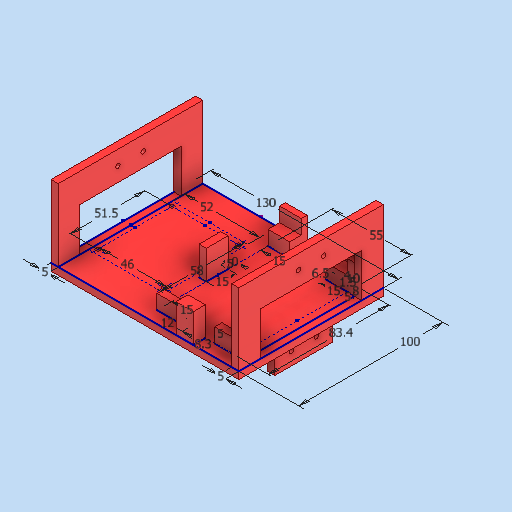
# Autodesk Inventor part: Chasis 2
Saved by Autodesk Inventor 2026.2 (Build 302298010, 298A)
## iProperties
Created: 2025-12-05
Part Number: Chasis 2
Material: Generic
Document SubType Name: Modeling
Designer: maxim
Density: 1 g/cm^3
Appearance: Light Red
Author: maxim
Autodesk Inventor part; units mm, degrees
ref_plane "YZ Plane" through (0, 0, 0) normal (1, 0, 0) x (0, 1, 0)
ref_plane "XZ Plane" through (0, 0, 0) normal (0, 1, 0) x (-1, 0, 0)
sketch "Sketch1" plane through (0, 0, 0) normal (0, 1, 0) x (-1, 0, 0)
  line L0 (0, 0) -> (-130, 0)
  line L1 (-130, 0) -> (-130, -100)
  line L2 (-130, -100) -> (0, -100)
  line L3 (0, -100) -> (0, 0)
  line L4 (-5, -21) -> (-57, -21) construction
  line L5 (-65, -21) -> (-65, -79) construction
  line L6 (-57, -79) -> (-5, -79) construction
  line L7 (-5, -79) -> (-5, -21) construction
  line L8 (-65, -91.7) -> (-120, -91.7) construction
  line L9 (-120, -91.7) -> (-120, -8.3) construction
  line L10 (-120, -8.3) -> (-65, -8.3) construction
  line L11 (-65, -8.3) -> (-65, -91.7) construction
  line L12 (-5, 0) -> (-5, -100)
  line L13 (-125, -100) -> (-125, 0)
  line L14 (-86.5, 0) -> (-98.5, 0)
  line L15 (-98.5, 0) -> (-98.5, -8.3)
  line L16 (-98.5, -8.3) -> (-86.5, -8.3)
  line L17 (-86.5, -8.3) -> (-86.5, 0)
  line L18 (-87.5, -100) -> (-97.5, -100)
  line L19 (-110, -93.2) -> (-120, -93.2)
  line L20 (-120, -93.2) -> (-120, -85.2)
  line L21 (-120, -85.2) -> (-125, -85.2)
  line L22 (-125, -85.2) -> (-125, -97.2)
  line L23 (-125, -97.2) -> (-110, -97.2)
  line L24 (-110, -97.2) -> (-110, -93.2)
  line L25 (-57, -79) -> (-57, -21) construction
  line L26 (-120, -8.3) -> (-105, -8.3)
  line L27 (-105, -8.3) -> (-105, -13.3)
  line L28 (-105, -13.3) -> (-120, -13.3)
  line L29 (-120, -13.3) -> (-120, -8.3)
  line L30 (-65, -8.3) -> (-80, -8.3)
  line L31 (-80, -8.3) -> (-80, -13.3)
  line L32 (-80, -13.3) -> (-65, -13.3)
  line L33 (-65, -13.3) -> (-65, -8.3)
  line L34 (-120, -91.7) -> (-105, -91.7)
  line L35 (-105, -91.7) -> (-105, -85.2)
  line L36 (-105, -85.2) -> (-120, -85.2)
  line L37 (-120, -85.2) -> (-120, -91.7)
  line L38 (-65, -91.7) -> (-80, -91.7)
  line L39 (-80, -91.7) -> (-80, -85.2)
  line L40 (-80, -85.2) -> (-65, -85.2)
  line L41 (-65, -85.2) -> (-65, -91.7)
  line L42 (-65, -42.5) -> (-60, -42.5)
  line L43 (-60, -42.5) -> (-60, -57.5)
  line L44 (-60, -57.5) -> (-65, -57.5)
  line L45 (-65, -57.5) -> (-65, -42.5)
  line L46 (-54, -75.75) -> (-8, -75.75) construction
  line L47 (-8, -75.75) -> (-8, -24.25) construction
  line L48 (-120, -91.7) -> (-105, -91.7)
  line L49 (-105, -91.7) -> (-105, -93.2)
  line L50 (-105, -93.2) -> (-120, -93.2)
  line L51 (-120, -93.2) -> (-120, -91.7)
  line L52 (-80, -91.7) -> (-65, -91.7)
  line L53 (-65, -91.7) -> (-65, -93.2)
  line L54 (-65, -93.2) -> (-80, -93.2)
  line L55 (-80, -93.2) -> (-80, -91.7)
  line L56 (-80, -93.2) -> (-65, -93.2)
  line L57 (-65, -93.2) -> (-65, -97.2)
  line L58 (-65, -97.2) -> (-80, -97.2)
  line L59 (-80, -97.2) -> (-80, -93.2)
  point P0 (0, -50)
  point P1 (-65, -50)
  point P2 (-65, -100)
  point P3 (-120, -50)
  point P4 (-120, -50)
  point P5 (-54, -24.25)
  point P6 (-92.5, -8.3)
  point P7 (-92.5, -8.3)
  point P8 (-86.5, 0)
  point P9 (-98.5, 0)
  point P10 (-45, -100)
  point P11 (-95, -100)
  point P12 (-92.5, -91.7)
  point P13 (-110, -95.2)
  point P14 (-115, -93.2)
  point P15 (-125, -85.2)
  point P16 (-125, -97.2)
  point P17 (-5, -50)
  point P18 (-57, -50)
  point P19 (-65, -50)
  point P20 (-31, -75.75)
  point P21 (-31, -79)
  point P22 (-8, -50)
  point P23 (-75, -93)
  point P24 (-65, -93)
  point P25 (-72.5, -97.2)
  point P26 (-65, -93.2)
  dimension "d0" = 100
  dimension "d1" = 130
  dimension "d2" = 52
  dimension "d3" = 58
  dimension "d5" = 55
  dimension "d6" = 83.4
  dimension "d10" = 5
  dimension "d11" = 5
  dimension "d16" = 12
  dimension "d17" = 8.3
  dimension "d88" = 10
  dimension "d89" = 5
  dimension "d90" = 4
  dimension "d92" = 8
  dimension "d93" = 1.5
  dimension "d101" = 15
  dimension "d102" = 15
  dimension "d103" = 6.5
  dimension "d104" = 5
  dimension "d105" = 15
  dimension "d111" = 0
  dimension "d112" = 15
  dimension "d113" = 5
  dimension "d116" = 46
  dimension "d117" = 51.5
  constraints: 120 end point, 24 parallel, 19 perpendicular, 18 midpoint, 14 horizontal, 11 point on line, 8 horizontal alignment, 6 vertical alignment, 3 coincident, 3 vertical
  measures "d0" distance of L0.end L1.end
  measures "d1" distance of L1.end L2.end
  measures "d2" distance of L6.start L6.end
  measures "d3" distance between parallel lines of L6 L4
  measures "d5" distance between parallel lines of L9 L11
  measures "d6" distance between parallel lines of L10 L8
  measures "d10" distance between parallel lines of L12 L3
  measures "d11" distance between parallel lines of L1 L13
  measures "d16" distance of L16.end L15.end
  measures "d17" distance between parallel lines of L14 L16
  measures "d88" distance from line of point (-110, -95.2) L20
  measures "d89" distance between parallel lines of L22 L20
  measures "d90" distance from line of L23 point (-115, -93.2)
  measures "d92" distance between parallel lines of L21 L19
  measures "d93" distance between parallel lines of L8 L19
  measures "d101" distance of L35.end L36.end
  measures "d102" distance of L39.end L40.end
  measures "d103" distance of L34.end L35.end
  measures "d104" distance of L26.end L27.end
  measures "d105" distance of L31.end L32.end
  measures "d111" distance between parallel lines of L45 L5
  measures "d112" distance of L42.end L43.end
  measures "d113" distance of L43.end L44.end
  measures "d116" distance of L47.end point (-54, -24.25)
  measures "d117" distance of L47.end L46.end
extrude "Extrusion2" add sketch "Sketch1" against normal blind 5 contours L3 L2 L12 L0 | L12 L2 L13 L23 L24 L50 L49 L35 L36 L21 L0 L15 L16 L17 | L17 L16 L15 L0 | L13 L2 L1 L0 | L21 L20 L19 L24 L23 L13 | L36 L35 L34 L20 | L34 L49 L50 L19 L20 | L26 L27 L28 L29 | L33 L32 L31 L30 | L53 L54 L55 L38 | L38 L39 L40 L41 | L57 L58 L59 L54 | L42 L43 L44 L45
hole "Hole1" at (8, 0, -75.75) at (8, 0, -24.25) at (54, 0, -75.75) at (54, 0, -24.25) direction (0, -1, 0) diameter 3.1 end through all
extrude "Extrusion5" add sketch "Sketch1" along normal blind 50 contours L3 L2 L12 L0 | L13 L2 L1 L0
extrude "Extrusion6" add sketch "Sketch1" along normal blind 20 contours L17 L16 L15 L0 | L21 L20 L19 L24 L23 L13
ref_plane "Work Plane1" through (65, -5, 0) normal (-1, 0, 0) x (0, 0, 1)
sketch "Sketch5" plane through (0, -5, 0) normal (0, -1, 0) x (1, 0, 0)
  line L0 (130, 0) -> (0, 0) projected
  line L1 (65, 0) -> (65, -100)
  line L2 (0, -100) -> (130, -100) projected
  line L3 (5, -30) -> (10, -30)
  line L4 (10, -30) -> (10, -70)
  line L5 (10, -70) -> (5, -70)
  line L6 (5, -70) -> (5, -30)
  line L7 (125, -30) -> (120, -30)
  line L8 (120, -30) -> (120, -70)
  line L9 (120, -70) -> (125, -70)
  line L10 (125, -70) -> (125, -30)
  point P0 (65, -50)
  point P1 (10, -50)
  dimension "d60" = 40
  dimension "d61" = 5
  dimension "d62" = 55
  constraints: 18 end point, 4 midpoint, 4 symmetric about line, 2 parallel, 1 horizontal, 1 horizontal alignment, 1 perpendicular
  measures "d60" distance of L3.end L4.end
  measures "d61" distance of L3.start L3.end
  measures "d62" distance between parallel lines of L1 L4
extrude "Extrusion9" add sketch "Sketch5" along normal blind 15
sketch "Sketch6" plane through (5, -5, -70) normal (-1, 0, 0) x (0, 0, 1)
  line L0 (11.25, -6) -> (28.75, -6) construction
  line L1 (70, 0) -> (-30, 0) projected
  line L2 (11.25, 36) -> (28.75, 36)
  point P0 (70, 5)
  point P1 (20, 0)
  point P2 (20, -6)
  dimension "d65" = 17.5
  dimension "d66" = 6
  dimension "d74" = 17.5
  constraints: 4 end point, 2 coincident, 2 horizontal, 2 midpoint, 1 vertical alignment
  measures "d65" distance of L0.start L0.end
  measures "d66" distance between parallel lines of L1 L0
  measures "d74" distance of L2.start L2.end
hole "Hole2" at (5, -11, -58.75) at (5, -11, -41.25) direction (1, 0, 0) diameter 3.1 end through all
sketch "Sketch7" plane through (0, -5, -100) normal (-1, 0, 0) x (0, 0, 1)
  line L0 (41.25, 45) -> (58.75, 45) construction
  line L1 (100, 0) -> (0, 0) projected
  line L2 (0, 55) -> (100, 55) projected
  point P0 (100, 5)
  point P1 (50, 45)
  point P2 (50, 0)
  dimension "d75" = 17.5
  dimension "d76" = 10
  constraints: 2 coincident, 2 end point, 2 midpoint, 1 horizontal, 1 vertical alignment
  measures "d75" distance of L0.start L0.end
  measures "d76" distance between parallel lines of L2 L0
hole "Hole3" at (0, 40, -58.75) at (0, 40, -41.25) direction (1, 0, 0) diameter 3.1 end through all
sketch "Sketch8" plane through (0, -5, -100) normal (-1, 0, 0) x (0, 0, 1)
  line L0 (100, 5) -> (0, 5) projected
  line L1 (15, 5) -> (85, 5)
  line L2 (85, 5) -> (85, 35)
  line L3 (85, 35) -> (15, 35)
  line L4 (15, 35) -> (15, 5)
  line L5 (0, 55) -> (100, 55) projected
  point P0 (14.8, 5)
  point P1 (50, 35)
  point P2 (50, 55)
  dimension "d95" = 70
  dimension "d96" = 30
  constraints: 8 end point, 2 midpoint, 2 parallel, 1 horizontal, 1 perpendicular, 1 point on line, 1 vertical alignment
  measures "d95" distance of L3.end L2.end
  measures "d96" distance between parallel lines of L0 L3
extrude "Extrusion10" cut sketch "Sketch8" against normal through all
extrude "Extrusion11" add sketch "Sketch1" along normal blind 10 contours L36 L35 L34 L20 | L34 L49 L50 L19 L20 | L26 L27 L28 L29 | L33 L32 L31 L30 | L53 L54 L55 L38 | L38 L39 L40 L41
extrude "Extrusion13" add sketch "Sketch1" along normal blind 20 contours L57 L58 L59 L54 | L42 L43 L44 L45
body "Solid1"
